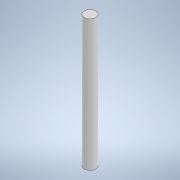
# Autodesk Inventor part: Eixo da roda
Saved by Autodesk Inventor 2021 (Build 250183000, 183)
## iProperties
Created: 2021-11-18
Part Number: Eixo da roda
Material: Generic
Document SubType Name: Modeling
Designer: Matheus
Density: 7.01169 g/cm^3
Appearance: Default
Mass: 1.7 g
Surface Area: 3.37407 cm^2
Volume: 0.242452 cm^3
Author: Matheus
Autodesk Inventor part; units mm, degrees
ref_plane "YZ Plane" through (0, 0, 0) normal (1, 0, 0) x (0, 1, 0)
ref_plane "XZ Plane" through (0, 0, 0) normal (0, 1, 0) x (-1, 0, 0)
ref_plane "XY Plane" through (0, 0, 0) normal (0, 0, 1) x (1, 0, 0)
sketch "Sketch1" plane through (0, 0, 0) normal (0, 1, 0) x (-1, 0, 0)
  circle A0 centre (0, 0) radius 1.5
  dimension "d0" = 3
  constraints: 1 centre point, 1 coincident
  measures "d0" diameter of A0
extrude "Extrusion1" add sketch "Sketch1" along normal blind 34.3
body "Solid1"
